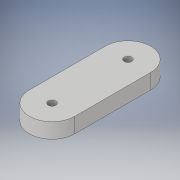
# Autodesk Inventor part: FirstChain
Saved by Autodesk Inventor 2019 (Build 230136000, 136)
## iProperties
Created: 2019-01-18
Part Number: FirstChain
Material: Generic
Document SubType Name: Modeling
Designer: mar22
Density: 1 g/cm^3
Appearance: Default
Author: mar22
Autodesk Inventor part; units mm, degrees
ref_plane "YZ Plane" through (0, 0, 0) normal (1, 0, 0) x (0, 1, 0)
ref_plane "XZ Plane" through (0, 0, 0) normal (0, 1, 0) x (-1, 0, 0)
ref_plane "XY Plane" through (0, 0, 0) normal (0, 0, 1) x (1, 0, 0)
sketch "Sketch1" plane through (0, 0, 0) normal (0, 1, 0) x (-1, 0, 0)
  line L0 (76.2, 0) -> (76.2, -127)
  line L1 (0, -127) -> (0, 0)
  arc A0 (0, -127) -> (76.2, -127) centre (38.1, -127) ccw
  arc A1 (76.2, 0) -> (0, 0) centre (38.1, 0) ccw
  circle A2 centre (38.1, 0) radius 6.35
  circle A3 centre (38.1, -127) radius 6.35
  dimension "d2" = 12.7
  dimension "d3" = 12.7
  dimension "d6" = 76.2
  constraints: 4 centre point, 4 end point, 4 point on circle, 2 coincident, 1 parallel
  measures "d2" diameter of A2
  measures "d3" diameter of A3
  measures "d6" distance between parallel lines of L1 L0
extrude "Extrusion1" add sketch "Sketch1" along normal blind 25.4
body "Solid1"
